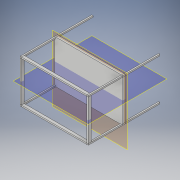
# Autodesk Inventor part: RobotFab Frame 2
Saved by Autodesk Inventor 2019 (Build 230136000, 136)
## iProperties
Created: 2021-01-25
Part Number: RobotFab Frame 2
Material: Generic
Document SubType Name: Modeling
Designer: Eric
Density: 1 g/cm^3
Appearance: Default
Author: Eric
Autodesk Inventor part; units mm, degrees
ref_plane "YZ Plane" through (0, 0, 0) normal (1, 0, 0) x (0, 1, 0)
ref_plane "XZ Plane" through (0, 0, 0) normal (0, 1, 0) x (-1, 0, 0)
ref_plane "XY Plane" through (0, 0, 0) normal (0, 0, 1) x (1, 0, 0)
sketch "Sketch1" plane through (0, 0, 0) normal (0, 0, 1) x (1, 0, 0)
  line L0 (0, 0) -> (40, 0)
  line L1 (40, 0) -> (40, -40)
  line L2 (40, -40) -> (0, -40)
  line L3 (0, -40) -> (0, 0)
  line L4 (40, 0) -> (1940, 0)
  line L5 (1940, 0) -> (1940, -40)
  line L6 (1940, -40) -> (1980, -40)
  line L7 (1980, -40) -> (1980, 0)
  line L8 (1980, 0) -> (1940, 0)
  line L9 (40, -40) -> (1940, -40)
  line L10 (0, -40) -> (0, -1209)
  line L11 (0, -1209) -> (40, -1209)
  line L12 (40, -1209) -> (40, -40)
  line L13 (0, -1209) -> (0, -1249)
  line L14 (0, -1249) -> (40, -1249)
  line L15 (40, -1249) -> (40, -1209)
  line L16 (1940, -1209) -> (1940, -1249)
  line L17 (1940, -1249) -> (40, -1249)
  line L18 (1940, -1209) -> (1980, -1209)
  line L19 (1980, -1209) -> (1980, -1249)
  line L20 (1980, -1249) -> (1940, -1249)
  line L21 (1940, -1209) -> (1940, -40)
  line L22 (1980, -40) -> (1980, -1209)
  line L23 (40, -1209) -> (1940, -1209)
  line L24 (40, -520) -> (1940, -520)
  line L25 (40, -560) -> (1940, -560)
  line L26 (490, -40) -> (490, -520)
  line L27 (530, -520) -> (530, -40)
  line L28 (830, -40) -> (830, -520)
  line L29 (870, -520) -> (870, -40)
  line L30 (1130, -40) -> (1130, -520)
  line L31 (1170, -520) -> (1170, -40)
  line L32 (1470, -40) -> (1470, -520)
  line L33 (1510, -520) -> (1510, -40)
  line L34 (240, -560) -> (240, -1209)
  line L35 (280, -1209) -> (280, -560)
  line L36 (600, -560) -> (600, -1209)
  line L37 (640, -1209) -> (640, -560)
  line L38 (900, -560) -> (900, -1209)
  line L39 (940, -1209) -> (940, -560)
  line L40 (1060, -560) -> (1060, -1209)
  line L41 (1100, -1209) -> (1100, -560)
  line L42 (1420, -560) -> (1420, -1209)
  line L43 (1460, -1209) -> (1460, -560)
  line L44 (1460, -749.4424) -> (1940, -749.4424)
  line L45 (1940, -749.4424) -> (1940, -789.4424)
  line L46 (1940, -789.4424) -> (1460, -789.4424)
  line L47 (1460, -789.4424) -> (1460, -749.4424)
  line L48 (1460, -984.7722) -> (1940, -984.7722)
  line L49 (1940, -984.7722) -> (1940, -1024.7722)
  line L50 (1940, -1024.7722) -> (1460, -1024.7722)
  line L51 (1460, -1024.7722) -> (1460, -984.7722)
  dimension "d15" = 40
  dimension "d16" = 480
  dimension "d17" = 649
  dimension "d11" = 40
  dimension "d12" = 40
  dimension "d13" = 40
  dimension "d14" = 40
  dimension "d18" = 40
  dimension "d19" = 40
  dimension "d20" = 40
  dimension "d21" = 40
  dimension "d22" = 470
  dimension "d23" = 340
  dimension "d24" = 490
  dimension "d25" = 340
  dimension "d26" = 40
  dimension "d27" = 40
  dimension "d28" = 40
  dimension "d29" = 40
  dimension "d30" = 40
  dimension "d31" = 200
  dimension "d32" = 880
  dimension "d35" = 480
  dimension "d51" = 40
  dimension "d52" = 40
  dimension "d53" = 1980
  dimension "d108" = 360
  dimension "d109" = 240
  constraints: 96 end point, 29 vertical, 9 horizontal, 6 point on line, 4 collinear, 48 other
  measures "d11" distance of L1.end L2.end
  measures "d12" distance of L0.end L1.end
  measures "d13" distance of L7.end L4.end
  measures "d14" distance of L10.end L13.end
  measures "d18" distance between parallel lines of L27 L26
  measures "d19" distance between parallel lines of L29 L28
  measures "d20" distance between parallel lines of L31 L30
  measures "d21" distance between parallel lines of L33 L32
  measures "d22" distance between parallel lines of L22 L33
  measures "d23" distance between parallel lines of L31 L33
  measures "d24" distance between parallel lines of L10 L26
  measures "d25" distance between parallel lines of L28 L26
  measures "d26" distance between parallel lines of L35 L34
  measures "d27" distance between parallel lines of L37 L36
  measures "d28" distance between parallel lines of L39 L38
  measures "d29" distance between parallel lines of L41 L40
  measures "d30" distance between parallel lines of L43 L42
  measures "d31" distance between parallel lines of L41 L38
  measures "d32" distance between parallel lines of L22 L41
  measures "d35" distance between parallel lines of L21 L43
  measures "d51" distance between parallel lines of L44 L46
  measures "d52" distance between parallel lines of L50 L48
  measures "d53" distance between parallel lines of L22 L10
  measures "d108" distance between parallel lines of L36 L34
  measures "d109" distance between parallel lines of L10 L34
extrude "Extrusion1" [suppressed]
extrude "Extrusion7" [suppressed]
extrude "Extrusion8" [suppressed]
extrude "Extrusion9" [suppressed]
extrude "Extrusion2" [suppressed]
extrude "Extrusion10" [suppressed]
extrude "Extrusion11" [suppressed]
extrude "Extrusion12" [suppressed]
extrude "Extrusion13" [suppressed]
extrude "Extrusion14" [suppressed]
extrude "Extrusion15" [suppressed]
extrude "Extrusion16" [suppressed]
extrude "Extrusion17" [suppressed]
extrude "Extrusion18" [suppressed]
extrude "Extrusion19" [suppressed]
extrude "Extrusion20" [suppressed]
extrude "Extrusion3" add sketch "Sketch1" along normal blind 1080 and the other way blind 1000 separate body contours L0 L1 L2 L3
extrude "Extrusion21" add sketch "Sketch1" along normal blind 1080 and the other way blind 1000 separate body contours L11 L15 L14 L13
extrude "Extrusion22" add sketch "Sketch1" along normal blind 1080 and the other way blind 1000 separate body contours L19 L20 L16 L18
extrude "Extrusion23" add sketch "Sketch1" along normal blind 1080 and the other way blind 1000 separate body contours L8 L7 L6 L5
sketch "Sketch2" plane through (0, 0, 1080) normal (0, 0, 1) x (1, 0, 0)
  line L0 (0, 0) -> (0, -40) projected
  line L1 (0, -40) -> (40, -40) projected
  line L2 (40, -40) -> (40, 0) projected
  line L3 (40, 0) -> (0, 0) projected
  line L4 (1940, 0) -> (1940, -40) projected
  line L5 (1940, -40) -> (1980, -40) projected
  line L6 (1980, -40) -> (1980, 0) projected
  line L7 (1980, 0) -> (1940, 0) projected
  line L8 (1940, -1209) -> (1940, -1249) projected
  line L9 (1940, -1249) -> (1980, -1249) projected
  line L10 (1980, -1249) -> (1980, -1209) projected
  line L11 (1980, -1209) -> (1940, -1209) projected
  line L12 (0, -1209) -> (0, -1249) projected
  line L13 (0, -1249) -> (40, -1249) projected
  line L14 (40, -1249) -> (40, -1209) projected
  line L15 (40, -1209) -> (0, -1209) projected
  line L16 (0, -1209) -> (40, -1209)
  line L17 (40, -1209) -> (40, -40)
  line L18 (40, -40) -> (0, -40)
  line L19 (0, -40) -> (0, -1209)
  line L20 (40, 0) -> (1940, 0)
  line L21 (1940, 0) -> (1940, -40)
  line L22 (1940, -40) -> (40, -40)
  line L23 (40, -40) -> (40, 0)
  line L24 (1940, -40) -> (1980, -40)
  line L25 (1980, -40) -> (1980, -1209)
  line L26 (1980, -1209) -> (1940, -1209)
  line L27 (1940, -1209) -> (1940, -40)
  line L28 (40, -1209) -> (1940, -1209)
  line L29 (1940, -1209) -> (1940, -1249)
  line L30 (1940, -1249) -> (40, -1249)
  line L31 (40, -1249) -> (40, -1209)
  line L32 (40, -1209) -> (0, -1209) projected
  line L33 (0, -1249) -> (40, -1249) projected
  line L34 (1940, -1209) -> (1940, -1249) projected
  line L35 (1980, -1209) -> (1940, -1209) projected
  line L36 (1940, -40) -> (1980, -40) projected
  line L37 (1940, 0) -> (1940, -40) projected
  line L38 (1980, 0) -> (1940, 0) projected
  line L39 (0, -40) -> (40, -40) projected
  constraints: 32 end point, 16 collinear
extrude "Extrusion4" add sketch "Sketch2" against normal blind 80 separate body contours L1 L17 L15 L19
extrude "Extrusion24" add sketch "Sketch2" against normal blind 80 separate body contours L28 L8 L30 L14
extrude "Extrusion25" add sketch "Sketch2" against normal blind 80 separate body contours L5 L25 L11 L27
extrude "Extrusion26" add sketch "Sketch2" against normal blind 80 separate body contours L20 L4 L22 L2
sketch "Sketch3" plane through (0, 0, 80) normal (0, 0, -1) x (-1, 0, 0)
  line L0 (-850, -1749) -> (-890, -1749)
  line L1 (-890, -1749) -> (-890, -1249)
  line L2 (-890, -1249) -> (-850, -1249)
  line L3 (-850, -1249) -> (-850, -1749)
  line L4 (-1110, -1749) -> (-1150, -1749)
  line L5 (-1150, -1749) -> (-1150, -1249)
  line L6 (-1150, -1249) -> (-1110, -1249)
  line L7 (-1110, -1249) -> (-1110, -1749)
  line L8 (-1940, -1249) -> (-40, -1249) construction
  point P0 (0, 0)
  point P1 (0, -1249)
  dimension "d44" = 40
  dimension "d45" = 40
  dimension "d46" = 300
  dimension "d48" = 500
  dimension "d105" = 850
  constraints: 16 end point, 4 horizontal, 2 collinear, 1 parallel, 1 vertical
  measures "d44" distance between parallel lines of L1 L3
  measures "d45" distance between parallel lines of L5 L7
  measures "d46" distance between parallel lines of L3 L5
  measures "d48" distance of L4.end L5.end
  measures "d105" distance from line of point (0, -1249) L3
extrude "Extrusion5" [suppressed]
extrude "Extrusion27" [suppressed]
ref_plane "Work Plane5" through (850, -874.5, 80) normal (0, -1, 0) x (-1, 0, 0)
ref_plane "Work Plane6" through (990, -1209, 0) normal (-1, 0, 0) x (0, 0, 1)
ref_plane "Work Plane7" through (0, 0, 40) normal (0, 0, 1) x (1, 0, 0)
ref_plane "Work Plane8" through (40, -624.5, 1080) normal (0, -1, 0) x (1, 0, 0)
extrude "Extrusion28" add sketch "Sketch1" along normal blind 80 separate body
equation "\"d15\" = d12"
equation "\"d11\" = d13"
equation "\"d14\" = d12"
equation "\"d18\" = d12"
equation "\"d19\" = d12"
equation "\"d20\" = d12"
equation "\"d21\" = d12"
equation "\"d26\" = d12"
equation "\"d27\" = d12"
equation "\"d28\" = d12"
equation "\"d29\" = d12"
equation "\"d30\" = d12"
equation "\"d32\" = d33"
equation "\"d51\" = d12"
equation "\"d52\" = d12"
equation "\"d45\" = d44"
equation "\"d33\" = 880"
body "Solid1"
body "Solid2"
body "Solid3"
body "Solid4"
body "Solid5"
body "Solid6"
body "Solid7"
body "Solid8"
body "Solid9"
body "Solid10"
body "Solid11"
body "Solid12"
body "Solid13"
body "Solid14"
body "Solid15"
body "Solid16"
body "Solid17"
body "Solid18"
body "Solid19"
body "Solid20"
body "Solid21"
body "Solid22"
body "Solid23"
body "Solid24"
body "Solid25"
body "Solid26"
body "Solid27"
